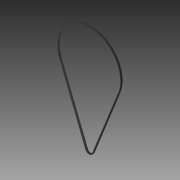
# Autodesk Inventor part: 2127_Timing Belt_V1
Saved by Autodesk Inventor 2020 (Build 240168000, 168)
## iProperties
Created: 2017-06-22
Part Number: 2127_Timing Belt_V1
Material: Rubber, Black
Document SubType Name: Modeling
Designer: MPI
Density: 0.93 g/cm^3
Appearance: Rubber - Black
Author: MPI
Autodesk Inventor part; units mm, degrees
ref_plane "YZ Plane" through (0, 0, 0) normal (1, 0, 0) x (0, 1, 0)
ref_plane "XZ Plane" through (0, 0, 0) normal (0, 1, 0) x (-1, 0, 0)
sketch "Sketch6" plane through (0, 0, 0) normal (0, 0, 1) x (1, 0, 0)
  arc A0 (213.8591, -85.1159) -> (-213.8591, -85.1159) centre (0, 0) ccw
  line L0 (213.8591, -85.1159) -> (26.0067, -557.1069)
  line L1 (-213.8591, -85.1159) -> (-26.0067, -557.1069)
  arc A1 (-26.0067, -557.1069) -> (26.0067, -557.1069) centre (0, -546.7562) ccw
  line L2 (23.9917, -556.3049) -> (211.8441, -84.3139)
  arc A2 (211.8441, -84.3139) -> (-211.8441, -84.3139) centre (0, 0) ccw
  line L3 (-211.8441, -84.3139) -> (-23.9917, -556.3049)
  arc A3 (-23.9917, -556.3049) -> (23.9917, -556.3049) centre (0, -546.7562) ccw
  dimension "d61" = 460.3496
  dimension "d63" = 55.9816
  dimension "d64" = 508
  dimension "d65" = 2.1688
  constraints: 8 end point, 8 point on circle, 4 centre point, 4 tangent, 1 coincident, 1 vertical alignment, 3 other
  measures "d61" diameter of A0
  measures "d63" diameter of A1
  measures "d64" distance of L0.start L0.end
  measures "d65" distance between parallel lines of L0 L2
extrude "Extrusion4" add sketch "Sketch6" along normal mid plane 12.7
sketch "Sketch7" plane through (0, 0, 6.35) normal (0, 0, 1) x (1, 0, 0)
  line L0 (-23.9917, -556.3049) -> (-211.8441, -84.3139) construction
  line L1 (-211.3488, -84.6559) -> (-210.0329, -84.6168)
  line L2 (-208.4776, -88.5246) -> (-209.4601, -89.4)
  line L3 (-215.1708, -88.9251) -> (-184.5764, -76.7485) construction
  line L4 (-209.5459, -84.9368) -> (-208.3436, -87.9575)
  arc A0 (-211.8441, -84.3139) -> (-211.3488, -84.6559) centre (-211.3639, -84.1482) ccw
  arc A1 (-209.5459, -84.9368) -> (-210.0329, -84.6168) centre (-210.0178, -85.1246) ccw
  arc A2 (-208.4776, -88.5246) -> (-208.3436, -87.9575) centre (-208.8156, -88.1454) ccw
  arc A3 (-209.4601, -89.4) -> (-209.5941, -89.9671) centre (-209.1221, -89.7793) ccw
  line L5 (-211.8441, -84.3139) -> (-209.5941, -89.9671)
  point P0 (-210.0414, -89.918)
  point P1 (-203.887, -84.4342)
  point P2 (-211.7038, -84.6665)
  point P3 (-211.8267, -84.3577)
  dimension "d68" = 40
  dimension "d69" = 20
  dimension "d70" = 1.905
  dimension "d71" = 0.508
  dimension "d72" = 0.508
  dimension "d73" = 3.2512
  dimension "d74" = 1.3158
  dimension "d75" = 1.3158
  constraints: 10 end point, 8 point on circle, 7 point on line, 6 tangent, 4 centre point, 2 equal radius, 1 parallel, 1 perpendicular
  measures "d68" angle of L2 L1
  measures "d69" angle of L3 L1
  measures "d70" distance between parallel lines of L0 L4
  measures "d71" radius of A0
  measures "d72" radius of A3
  measures "d73" distance of L4.start L4.end
  measures "d74" distance of L2.start L2.end
  measures "d75" horizontal distance of L1.start L1.end
extrude "Extrusion5" add sketch "Sketch7" against normal up to surface (12.7 mm away)
pattern_linear "Rectangular Pattern3" count 55 spacing 9.525 along (0.3697882, -0.9291161, 0) of "Extrusion5"
ref_plane "Work Plane3" through (0, -622.4504, -6.35) normal (-1, 0, 0) x (0, 0, -1)
mirror "Mirror3" about plane through (0, -622.4504, -6.35) normal (-1, 0, 0) of "Extrusion5", "Rectangular Pattern3"
pattern_circular "Circular Pattern1" count 57 over 217.7 about axis through (0, 0, 0) along (0, 0, -1) of "Extrusion5"
body "Solid2"
